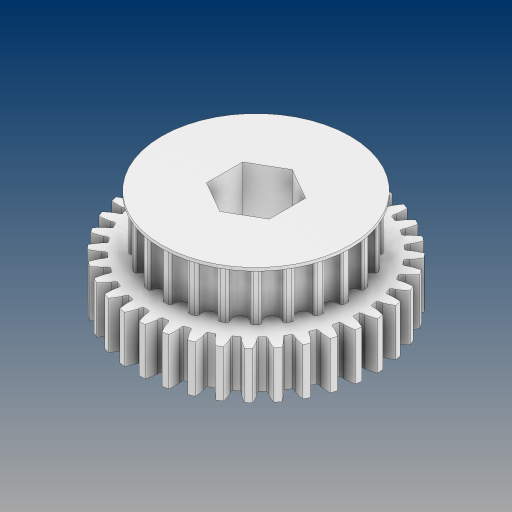
# Autodesk Inventor part: SHOT_005_36TGear-24TPulley
Saved by Autodesk Inventor 2024.3 (Build 283343000, 343)
## iProperties
Created: 2024-08-09
Part Number: SHOT_005_36TGear-24TPulley
Material: ABS Plastic
Document SubType Name: Modeling
Designer: Kenji
Density: 1.06 g/cm^3
Appearance: Smooth - White
Author: Kenji
Autodesk Inventor part; units mm, degrees
(part 1 of 2)
ref_plane "YZ Plane" through (0, 0, 0) normal (1, 0, 0) x (0, 1, 0)
ref_plane "XZ Plane" through (0, 0, 0) normal (0, 1, 0) x (-1, 0, 0)
ref_plane "XY Plane" through (0, 0, 0) normal (0, 0, 1) x (1, 0, 0)
sketch "Sketch1" plane through (0, 0, 0) normal (0, 1, 0) x (-1, 0, 0)
  circle A0 centre (0, 0) radius 22.86 construction
  circle A1 centre (0, 0) radius 24.13 construction
  line L0 (0, 0) -> (22.86, 0) construction
  line L1 (0, 0) -> (21.4269, 5.5414) construction
  line L2 (21.4269, 5.5414) -> (22.86, 0) construction
  arc A2 (21.4269, 5.5414) -> (20.1275, 9.2034) centre (0, 0) ccw construction
  arc A3 (22.1315, -0.1227) -> (21.4269, 5.5414) centre (0, 0) ccw construction
  line L3 (22.86, 0) -> (22.1315, -0.1227) construction
  line L4 (20.1275, 9.2034) -> (24.1256, 0.4597) construction
  line L5 (21.2725, 11.3902) -> (21.2725, -11.3902) construction
  line L6 (22.1315, -0.1227) -> (21.2725, -0.3449) construction
  line L7 (23.1177, 6.9159) -> (18.5715, -15.4064) construction
  line L8 (22.1315, -0.1227) -> (21.6794, -0.1463) construction
  line L9 (21.6794, -0.1463) -> (21.2725, -0.3449) construction
  line L10 (23.4095, 5.8526) -> (17.8483, -16.2387) construction
  line L11 (22.1315, -0.1227) -> (21.9049, -0.1242) construction
  line L12 (21.9049, -0.1242) -> (21.6794, -0.1463) construction
  line L13 (22.6036, 8.4459) -> (19.5599, -14.1303) construction
  line L14 (21.6794, -0.1463) -> (21.4414, -0.1748) construction
  line L15 (21.4414, -0.1748) -> (21.2725, -0.3449) construction
  line L16 (0, 0) -> (21.255, -0.928) construction
  arc A4 (21.255, -0.928) -> (21.2725, -0.3449) centre (0, 0) ccw
  arc A5 (21.2216, -1.5105) -> (21.255, -0.928) centre (0, 0) ccw
  line L17 (24.1256, 0.4597) -> (22.86, 0) construction
  line L18 (22.86, 0) -> (22.1315, -0.1227) construction
  spline S0 degree 2 poles (24.1256, 0.4597) (22.86, 0) (22.1315, -0.1227) knots 1 1 1 2 2 2
  line L19 (22.1315, -0.1227) -> (21.9049, -0.1242) construction
  line L20 (21.9049, -0.1242) -> (21.6794, -0.1463) construction
  line L21 (21.6794, -0.1463) -> (21.4414, -0.1748) construction
  line L22 (21.4414, -0.1748) -> (21.2725, -0.3449) construction
  spline S1 degree 4 poles (22.1315, -0.1227) (21.9049, -0.1242) (21.6794, -0.1463) (21.4414, -0.1748) (21.2725, -0.3449) knots 1 1 1 1 1 2 2 2 2 2
  arc A6 (21.2216, -1.5105) -> (21.255, -0.928) centre (0, 0) ccw
  line L23 (23.9937, -2.5606) -> (22.773, -1.9924) construction
  line L24 (22.773, -1.9924) -> (22.058, -1.8066) construction
  spline S2 degree 2 poles (23.9937, -2.5606) (22.773, -1.9924) (22.058, -1.8066) knots 1 1 1 2 2 2
  line L25 (22.058, -1.8066) -> (21.8324, -1.7854) construction
  line L26 (21.8324, -1.7854) -> (21.6096, -1.7437) construction
  line L27 (21.6096, -1.7437) -> (21.375, -1.6946) construction
  line L28 (21.375, -1.6946) -> (21.2216, -1.5105) construction
  spline S3 degree 4 poles (22.058, -1.8066) (21.8324, -1.7854) (21.6096, -1.7437) (21.375, -1.6946) (21.2216, -1.5105) knots 1 1 1 1 1 2 2 2 2 2
  line L29 (23.6793, 4.6421) -> (22.5127, 3.9696) construction
  spline S4 degree 2 poles (23.6793, 4.6421) (22.5127, 3.9696) (21.8166, 3.7222) knots 1 1 1 2 2 2
  line L30 (22.5127, 3.9696) -> (21.8166, 3.7222) construction
  spline S5 degree 2 poles (24.0739, 1.6447) (22.773, 1.9924) (22.0366, 2.0511) knots 1 1 1 2 2 2
  line L31 (24.0739, 1.6447) -> (22.773, 1.9924) construction
  line L32 (22.773, 1.9924) -> (22.0366, 2.0511) construction
  line L33 (22.0366, 2.0511) -> (21.8107, 2.0328) construction
  spline S6 degree 4 poles (22.0366, 2.0511) (21.8107, 2.0328) (21.5841, 2.0352) (21.3446, 2.0429) (21.1615, 2.1976) knots 1 1 1 1 1 2 2 2 2 2
  line L34 (21.8107, 2.0328) -> (21.5841, 2.0352) construction
  line L35 (21.5841, 2.0352) -> (21.3446, 2.0429) construction
  line L36 (21.3446, 2.0429) -> (21.1615, 2.1976) construction
  arc A7 (21.1615, 2.1976) -> (21.0933, 2.777) centre (0, 0) ccw
  arc A8 (21.0933, 2.777) -> (21.0092, 3.3543) centre (0, 0) ccw
  spline S7 degree 4 poles (21.8166, 3.7222) (21.5937, 3.6815) (21.3754, 3.6205) (21.146, 3.5511) (21.0092, 3.3543) knots 1 1 1 1 1 2 2 2 2 2
  line L37 (21.8166, 3.7222) -> (21.5937, 3.6815) construction
  line L38 (21.5937, 3.6815) -> (21.3754, 3.6205) construction
  line L39 (21.3754, 3.6205) -> (21.146, 3.5511) construction
  line L40 (21.146, 3.5511) -> (21.0092, 3.3543) construction
  line L41 (22.5134, 8.6834) -> (21.4814, 7.8186) construction
  spline S8 degree 2 poles (22.5134, 8.6834) (21.4814, 7.8186) (20.8388, 7.4541) knots 1 1 1 2 2 2
  line L42 (21.4814, 7.8186) -> (20.8388, 7.4541) construction
  spline S9 degree 2 poles (23.4225, 5.8001) (22.0811, 5.9166) (21.3456, 5.8466) knots 1 1 1 2 2 2
  line L43 (23.4225, 5.8001) -> (22.0811, 5.9166) construction
  line L44 (22.0811, 5.9166) -> (21.3456, 5.8466) construction
  line L45 (21.3456, 5.8466) -> (21.1264, 5.7894) construction
  spline S10 degree 4 poles (21.3456, 5.8466) (21.1264, 5.7894) (20.9028, 5.7524) (20.6656, 5.7183) (20.4584, 5.8389) knots 1 1 1 1 1 2 2 2 2 2
  line L46 (21.1264, 5.7894) -> (20.9028, 5.7524) construction
  line L47 (20.9028, 5.7524) -> (20.6656, 5.7183) construction
  line L48 (20.6656, 5.7183) -> (20.4584, 5.8389) construction
  arc A9 (20.4584, 5.8389) -> (20.2906, 6.3976) centre (0, 0) ccw
  arc A10 (20.2906, 6.3976) -> (20.1076, 6.9515) centre (0, 0) ccw
  spline S11 degree 4 poles (20.8388, 7.4541) (20.6264, 7.3752) (20.422, 7.2773) (20.2081, 7.1691) (20.1076, 6.9515) knots 1 1 1 1 1 2 2 2 2 2
  line L49 (20.8388, 7.4541) -> (20.6264, 7.3752) construction
  line L50 (20.6264, 7.3752) -> (20.422, 7.2773) construction
  line L51 (20.422, 7.2773) -> (20.2081, 7.1691) construction
  line L52 (20.2081, 7.1691) -> (20.1076, 6.9515) construction
  line L53 (20.6635, 12.4609) -> (19.7973, 11.43) construction
  spline S12 degree 2 poles (20.6635, 12.4609) (19.7973, 11.43) (19.2278, 10.9595) knots 1 1 1 2 2 2
  line L54 (19.7973, 11.43) -> (19.2278, 10.9595) construction
  spline S13 degree 2 poles (22.0595, 9.7793) (20.7182, 9.6611) (20.0061, 9.4644) knots 1 1 1 2 2 2
  line L55 (22.0595, 9.7793) -> (20.7182, 9.6611) construction
  line L56 (20.7182, 9.6611) -> (20.0061, 9.4644) construction
  line L57 (20.0061, 9.4644) -> (19.8001, 9.37) construction
  spline S14 degree 4 poles (20.0061, 9.4644) (19.8001, 9.37) (19.5864, 9.2947) (19.3586, 9.2199) (19.1337, 9.3027) knots 1 1 1 1 1 2 2 2 2 2
  line L58 (19.8001, 9.37) -> (19.5864, 9.2947) construction
  line L59 (19.5864, 9.2947) -> (19.3586, 9.2199) construction
  line L60 (19.3586, 9.2199) -> (19.1337, 9.3027) construction
  arc A11 (19.1337, 9.3027) -> (18.8714, 9.8238) centre (0, 0) ccw
  arc A12 (18.8714, 9.8238) -> (18.595, 10.3376) centre (0, 0) ccw
  spline S15 degree 4 poles (19.2278, 10.9595) (19.0323, 10.8449) (18.8481, 10.713) (18.6562, 10.5693) (18.595, 10.3376) knots 1 1 1 1 1 2 2 2 2 2
  line L61 (19.2278, 10.9595) -> (19.0323, 10.8449) construction
  line L62 (19.0323, 10.8449) -> (18.8481, 10.713) construction
  line L63 (18.8481, 10.713) -> (18.6562, 10.5693) construction
  line L64 (18.6562, 10.5693) -> (18.595, 10.3376) construction
  line L65 (18.1858, 15.8598) -> (17.5118, 14.6941) construction
  spline S16 degree 2 poles (18.1858, 15.8598) (17.5118, 14.6941) (17.0326, 14.1319) knots 1 1 1 2 2 2
  line L66 (17.5118, 14.6941) -> (17.0326, 14.1319) construction
  spline S17 degree 2 poles (20.0262, 13.4613) (18.7258, 13.112) (18.0587, 12.7946) knots 1 1 1 2 2 2
  line L67 (20.0262, 13.4613) -> (18.7258, 13.112) construction
  line L68 (18.7258, 13.112) -> (18.0587, 12.7946) construction
  line L69 (18.0587, 12.7946) -> (17.8722, 12.6659) construction
  spline S18 degree 4 poles (18.0587, 12.7946) (17.8722, 12.6659) (17.6748, 12.5546) (17.4635, 12.4415) (17.2276, 12.4839) knots 1 1 1 1 1 2 2 2 2 2
  line L70 (17.8722, 12.6659) -> (17.6748, 12.5546) construction
  line L71 (17.6748, 12.5546) -> (17.4635, 12.4415) construction
  line L72 (17.4635, 12.4415) -> (17.2276, 12.4839) construction
  arc A13 (17.2276, 12.4839) -> (16.8788, 12.9516) centre (0, 0) ccw
  arc A14 (16.8788, 12.9516) -> (16.5174, 13.4095) centre (0, 0) ccw
  spline S19 degree 4 poles (17.0326, 14.1319) (16.86, 13.9851) (16.7014, 13.8232) (16.5374, 13.6484) (16.5174, 13.4095) knots 1 1 1 1 1 2 2 2 2 2
  line L73 (17.0326, 14.1319) -> (16.86, 13.9851) construction
  line L74 (16.86, 13.9851) -> (16.7014, 13.8232) construction
  line L75 (16.7014, 13.8232) -> (16.5374, 13.6484) construction
  line L76 (16.5374, 13.6484) -> (16.5174, 13.4095) construction
  line L77 (15.1555, 18.7768) -> (14.6941, 17.5118) construction
  spline S20 degree 2 poles (15.1555, 18.7768) (14.6941, 17.5118) (14.3199, 16.8748) knots 1 1 1 2 2 2
  line L78 (14.6941, 17.5118) -> (14.3199, 16.8748) construction
  spline S21 degree 2 poles (17.3845, 16.7343) (16.1645, 16.1645) (15.5626, 15.7361) knots 1 1 1 2 2 2
  line L79 (17.3845, 16.7343) -> (16.1645, 16.1645) construction
  line L80 (16.1645, 16.1645) -> (15.5626, 15.7361) construction
  line L81 (15.5626, 15.7361) -> (15.4013, 15.5769) construction
  spline S22 degree 4 poles (15.5626, 15.7361) (15.4013, 15.5769) (15.2262, 15.4331) (15.0378, 15.2849) (14.7981, 15.2858) knots 1 1 1 1 1 2 2 2 2 2
  line L82 (15.4013, 15.5769) -> (15.2262, 15.4331) construction
  line L83 (15.2262, 15.4331) -> (15.0378, 15.2849) construction
  line L84 (15.0378, 15.2849) -> (14.7981, 15.2858) construction
  arc A15 (14.7981, 15.2858) -> (14.3734, 15.6858) centre (0, 0) ccw
  arc A16 (14.3734, 15.6858) -> (13.9379, 16.074) centre (0, 0) ccw
  spline S23 degree 4 poles (14.3199, 16.8748) (14.1753, 16.7003) (14.0473, 16.5133) (13.9162, 16.3127) (13.9379, 16.074) knots 1 1 1 1 1 2 2 2 2 2
  line L85 (14.3199, 16.8748) -> (14.1753, 16.7003) construction
  line L86 (14.1753, 16.7003) -> (14.0473, 16.5133) construction
  line L87 (14.0473, 16.5133) -> (13.9162, 16.3127) construction
  line L88 (13.9162, 16.3127) -> (13.9379, 16.074) construction
  line L89 (11.6647, 21.1233) -> (11.43, 19.7973) construction
  spline S24 degree 2 poles (11.6647, 21.1233) (11.43, 19.7973) (11.172, 19.1051) knots 1 1 1 2 2 2
  line L90 (11.43, 19.7973) -> (11.172, 19.1051) construction
  spline S25 degree 2 poles (14.2145, 19.4989) (13.112, 18.7258) (12.5936, 18.1995) knots 1 1 1 2 2 2
  line L91 (14.2145, 19.4989) -> (13.112, 18.7258) construction
  line L92 (13.112, 18.7258) -> (12.5936, 18.1995) construction
  line L93 (12.5936, 18.1995) -> (12.4624, 18.0147) construction
  spline S26 degree 4 poles (12.5936, 18.1995) (12.4624, 18.0147) (12.3149, 17.8426) (12.1551, 17.664) (11.9189, 17.6232) knots 1 1 1 1 1 2 2 2 2 2
  line L94 (12.4624, 18.0147) -> (12.3149, 17.8426) construction
  line L95 (12.3149, 17.8426) -> (12.1551, 17.664) construction
  line L96 (12.1551, 17.664) -> (11.9189, 17.6232) construction
  arc A17 (11.9189, 17.6232) -> (11.4312, 17.9434) centre (0, 0) ccw
  arc A18 (11.4312, 17.9434) -> (10.9349, 18.2501) centre (0, 0) ccw
  spline S27 degree 4 poles (11.172, 19.1051) (11.06, 18.9081) (10.9664, 18.7017) (10.8721, 18.4814) (10.9349, 18.2501) knots 1 1 1 1 1 2 2 2 2 2
  line L97 (11.172, 19.1051) -> (11.06, 18.9081) construction
  line L98 (11.06, 18.9081) -> (10.9664, 18.7017) construction
  line L99 (10.9664, 18.7017) -> (10.8721, 18.4814) construction
  line L100 (10.8721, 18.4814) -> (10.9349, 18.2501) construction
  line L101 (7.8195, 22.8279) -> (7.8186, 21.4814) construction
  spline S28 degree 2 poles (7.8195, 22.8279) (7.8186, 21.4814) (7.6847, 20.7548) knots 1 1 1 2 2 2
  line L102 (7.8186, 21.4814) -> (7.6847, 20.7548) construction
  spline S29 degree 2 poles (10.6126, 21.671) (9.6611, 20.7182) (9.242, 20.1098) knots 1 1 1 2 2 2
  line L103 (10.6126, 21.671) -> (9.6611, 20.7182) construction
  line L104 (9.6611, 20.7182) -> (9.242, 20.1098) construction
  line L105 (9.242, 20.1098) -> (9.1449, 19.9051) construction
  spline S30 degree 4 poles (9.242, 20.1098) (9.1449, 19.9051) (9.0295, 19.71) (8.9031, 19.5064) (8.6776, 19.4252) knots 1 1 1 1 1 2 2 2 2 2
  line L106 (9.1449, 19.9051) -> (9.0295, 19.71) construction
  line L107 (9.0295, 19.71) -> (8.9031, 19.5064) construction
  line L108 (8.9031, 19.5064) -> (8.6776, 19.4252) construction
  arc A19 (8.6776, 19.4252) -> (8.1417, 19.6558) centre (0, 0) ccw
  arc A20 (8.1417, 19.6558) -> (7.5997, 19.8717) centre (0, 0) ccw
  spline S31 degree 4 poles (7.6847, 20.7548) (7.6086, 20.5414) (7.5523, 20.3219) (7.4976, 20.0885) (7.5997, 19.8717) knots 1 1 1 1 1 2 2 2 2 2
  line L109 (7.6847, 20.7548) -> (7.6086, 20.5414) construction
  line L110 (7.6086, 20.5414) -> (7.5523, 20.3219) construction
  line L111 (7.5523, 20.3219) -> (7.4976, 20.0885) construction
  line L112 (7.4976, 20.0885) -> (7.5997, 19.8717) construction
  line L113 (3.7366, 23.8389) -> (3.9696, 22.5127) construction
  spline S32 degree 2 poles (3.7366, 23.8389) (3.9696, 22.5127) (3.9639, 21.774) knots 1 1 1 2 2 2
  line L114 (3.9696, 22.5127) -> (3.9639, 21.774) construction
  spline S33 degree 2 poles (6.6882, 23.1846) (5.9166, 22.0811) (5.6095, 21.4092) knots 1 1 1 2 2 2
  line L115 (6.6882, 23.1846) -> (5.9166, 22.0811) construction
  line L116 (5.9166, 22.0811) -> (5.6095, 21.4092) construction
  line L117 (5.6095, 21.4092) -> (5.5495, 21.1907) construction
  spline S34 degree 4 poles (5.6095, 21.4092) (5.5495, 21.1907) (5.4697, 20.9785) (5.3806, 20.756) (5.1726, 20.6369) knots 1 1 1 1 1 2 2 2 2 2
  line L118 (5.5495, 21.1907) -> (5.4697, 20.9785) construction
  line L119 (5.4697, 20.9785) -> (5.3806, 20.756) construction
  line L120 (5.3806, 20.756) -> (5.1726, 20.6369) construction
  arc A21 (5.1726, 20.6369) -> (4.6048, 20.771) centre (0, 0) ccw
  arc A22 (4.6048, 20.771) -> (4.0336, 20.8894) centre (0, 0) ccw
  spline S35 degree 4 poles (3.9639, 21.774) (3.926, 21.5506) (3.9087, 21.3246) (3.8954, 21.0853) (4.0336, 20.8894) knots 1 1 1 1 1 2 2 2 2 2
  line L121 (3.9639, 21.774) -> (3.926, 21.5506) construction
  line L122 (3.926, 21.5506) -> (3.9087, 21.3246) construction
  line L123 (3.9087, 21.3246) -> (3.8954, 21.0853) construction
  line L124 (3.8954, 21.0853) -> (4.0336, 20.8894) construction
  line L125 (-0.4597, 24.1256) -> (0, 22.86) construction
  spline S36 degree 2 poles (-0.4597, 24.1256) (0, 22.86) (0.1227, 22.1315) knots 1 1 1 2 2 2
  line L126 (0, 22.86) -> (0.1227, 22.1315) construction
  spline S37 degree 2 poles (2.5606, 23.9937) (1.9924, 22.773) (1.8066, 22.058) knots 1 1 1 2 2 2
  line L127 (2.5606, 23.9937) -> (1.9924, 22.773) construction
  line L128 (1.9924, 22.773) -> (1.8066, 22.058) construction
  line L129 (1.8066, 22.058) -> (1.7854, 21.8324) construction
  spline S38 degree 4 poles (1.8066, 22.058) (1.7854, 21.8324) (1.7437, 21.6096) (1.6946, 21.375) (1.5105, 21.2216) knots 1 1 1 1 1 2 2 2 2 2
  line L130 (1.7854, 21.8324) -> (1.7437, 21.6096) construction
  line L131 (1.7437, 21.6096) -> (1.6946, 21.375) construction
  line L132 (1.6946, 21.375) -> (1.5105, 21.2216) construction
  arc A23 (1.5105, 21.2216) -> (0.928, 21.255) centre (0, 0) ccw
  arc A24 (0.928, 21.255) -> (0.3449, 21.2725) centre (0, 0) ccw
  spline S39 degree 4 poles (0.1227, 22.1315) (0.1242, 21.9049) (0.1463, 21.6794) (0.1748, 21.4414) (0.3449, 21.2725) knots 1 1 1 1 1 2 2 2 2 2
  line L133 (0.1227, 22.1315) -> (0.1242, 21.9049) construction
  line L134 (0.1242, 21.9049) -> (0.1463, 21.6794) construction
  line L135 (0.1463, 21.6794) -> (0.1748, 21.4414) construction
  line L136 (0.1748, 21.4414) -> (0.3449, 21.2725) construction
  line L137 (-4.6421, 23.6793) -> (-3.9696, 22.5127) construction
  spline S40 degree 2 poles (-4.6421, 23.6793) (-3.9696, 22.5127) (-3.7222, 21.8166) knots 1 1 1 2 2 2
  line L138 (-3.9696, 22.5127) -> (-3.7222, 21.8166) construction
  spline S41 degree 2 poles (-1.6447, 24.0739) (-1.9924, 22.773) (-2.0511, 22.0366) knots 1 1 1 2 2 2
  line L139 (-1.6447, 24.0739) -> (-1.9924, 22.773) construction
  line L140 (-1.9924, 22.773) -> (-2.0511, 22.0366) construction
  line L141 (-2.0511, 22.0366) -> (-2.0328, 21.8107) construction
  spline S42 degree 4 poles (-2.0511, 22.0366) (-2.0328, 21.8107) (-2.0352, 21.5841) (-2.0429, 21.3446) (-2.1976, 21.1615) knots 1 1 1 1 1 2 2 2 2 2
  line L142 (-2.0328, 21.8107) -> (-2.0352, 21.5841) construction
  line L143 (-2.0352, 21.5841) -> (-2.0429, 21.3446) construction
  line L144 (-2.0429, 21.3446) -> (-2.1976, 21.1615) construction
  arc A25 (-2.1976, 21.1615) -> (-2.777, 21.0933) centre (0, 0) ccw
  arc A26 (-2.777, 21.0933) -> (-3.3543, 21.0092) centre (0, 0) ccw
  spline S43 degree 4 poles (-3.7222, 21.8166) (-3.6815, 21.5937) (-3.6205, 21.3754) (-3.5511, 21.146) (-3.3543, 21.0092) knots 1 1 1 1 1 2 2 2 2 2
  line L145 (-3.7222, 21.8166) -> (-3.6815, 21.5937) construction
  line L146 (-3.6815, 21.5937) -> (-3.6205, 21.3754) construction
  line L147 (-3.6205, 21.3754) -> (-3.5511, 21.146) construction
  line L148 (-3.5511, 21.146) -> (-3.3543, 21.0092) construction
  line L149 (-8.6834, 22.5134) -> (-7.8186, 21.4814) construction
  spline S44 degree 2 poles (-8.6834, 22.5134) (-7.8186, 21.4814) (-7.4541, 20.8388) knots 1 1 1 2 2 2
  line L150 (-7.8186, 21.4814) -> (-7.4541, 20.8388) construction
  spline S45 degree 2 poles (-5.8001, 23.4225) (-5.9166, 22.0811) (-5.8466, 21.3456) knots 1 1 1 2 2 2
  line L151 (-5.8001, 23.4225) -> (-5.9166, 22.0811) construction
  line L152 (-5.9166, 22.0811) -> (-5.8466, 21.3456) construction
  line L153 (-5.8466, 21.3456) -> (-5.7894, 21.1264) construction
  spline S46 degree 4 poles (-5.8466, 21.3456) (-5.7894, 21.1264) (-5.7524, 20.9028) (-5.7183, 20.6656) (-5.8389, 20.4584) knots 1 1 1 1 1 2 2 2 2 2
  line L154 (-5.7894, 21.1264) -> (-5.7524, 20.9028) construction
  line L155 (-5.7524, 20.9028) -> (-5.7183, 20.6656) construction
  line L156 (-5.7183, 20.6656) -> (-5.8389, 20.4584) construction
  arc A27 (-5.8389, 20.4584) -> (-6.3976, 20.2906) centre (0, 0) ccw
  arc A28 (-6.3976, 20.2906) -> (-6.9515, 20.1076) centre (0, 0) ccw
  spline S47 degree 4 poles (-7.4541, 20.8388) (-7.3752, 20.6264) (-7.2773, 20.422) (-7.1691, 20.2081) (-6.9515, 20.1076) knots 1 1 1 1 1 2 2 2 2 2
  line L157 (-7.4541, 20.8388) -> (-7.3752, 20.6264) construction
  line L158 (-7.3752, 20.6264) -> (-7.2773, 20.422) construction
  line L159 (-7.2773, 20.422) -> (-7.1691, 20.2081) construction
  line L160 (-7.1691, 20.2081) -> (-6.9515, 20.1076) construction
  line L161 (-12.4609, 20.6635) -> (-11.43, 19.7973) construction
  spline S48 degree 2 poles (-12.4609, 20.6635) (-11.43, 19.7973) (-10.9595, 19.2278) knots 1 1 1 2 2 2
  line L162 (-11.43, 19.7973) -> (-10.9595, 19.2278) construction
  spline S49 degree 2 poles (-9.7793, 22.0595) (-9.6611, 20.7182) (-9.4644, 20.0061) knots 1 1 1 2 2 2
  line L163 (-9.7793, 22.0595) -> (-9.6611, 20.7182) construction
  line L164 (-9.6611, 20.7182) -> (-9.4644, 20.0061) construction
  line L165 (-9.4644, 20.0061) -> (-9.37, 19.8001) construction
  spline S50 degree 4 poles (-9.4644, 20.0061) (-9.37, 19.8001) (-9.2947, 19.5864) (-9.2199, 19.3586) (-9.3027, 19.1337) knots 1 1 1 1 1 2 2 2 2 2
  line L166 (-9.37, 19.8001) -> (-9.2947, 19.5864) construction
  line L167 (-9.2947, 19.5864) -> (-9.2199, 19.3586) construction
  line L168 (-9.2199, 19.3586) -> (-9.3027, 19.1337) construction
  arc A29 (-9.3027, 19.1337) -> (-9.8238, 18.8714) centre (0, 0) ccw
  arc A30 (-9.8238, 18.8714) -> (-10.3376, 18.595) centre (0, 0) ccw
  spline S51 degree 4 poles (-10.9595, 19.2278) (-10.8449, 19.0323) (-10.713, 18.8481) (-10.5693, 18.6562) (-10.3376, 18.595) knots 1 1 1 1 1 2 2 2 2 2
  line L169 (-10.9595, 19.2278) -> (-10.8449, 19.0323) construction
  line L170 (-10.8449, 19.0323) -> (-10.713, 18.8481) construction
  line L171 (-10.713, 18.8481) -> (-10.5693, 18.6562) construction
  line L172 (-10.5693, 18.6562) -> (-10.3376, 18.595) construction
  line L173 (-15.8598, 18.1858) -> (-14.6941, 17.5118) construction
  spline S52 degree 2 poles (-15.8598, 18.1858) (-14.6941, 17.5118) (-14.1319, 17.0326) knots 1 1 1 2 2 2
  line L174 (-14.6941, 17.5118) -> (-14.1319, 17.0326) construction
  spline S53 degree 2 poles (-13.4613, 20.0262) (-13.112, 18.7258) (-12.7946, 18.0587) knots 1 1 1 2 2 2
  line L175 (-13.4613, 20.0262) -> (-13.112, 18.7258) construction
  line L176 (-13.112, 18.7258) -> (-12.7946, 18.0587) construction
  line L177 (-12.7946, 18.0587) -> (-12.6659, 17.8722) construction
  spline S54 degree 4 poles (-12.7946, 18.0587) (-12.6659, 17.8722) (-12.5546, 17.6748) (-12.4415, 17.4635) (-12.4839, 17.2276) knots 1 1 1 1 1 2 2 2 2 2
  line L178 (-12.6659, 17.8722) -> (-12.5546, 17.6748) construction
  line L179 (-12.5546, 17.6748) -> (-12.4415, 17.4635) construction
  line L180 (-12.4415, 17.4635) -> (-12.4839, 17.2276) construction
  arc A31 (-12.4839, 17.2276) -> (-12.9516, 16.8788) centre (0, 0) ccw
  arc A32 (-12.9516, 16.8788) -> (-13.4095, 16.5174) centre (0, 0) ccw
  spline S55 degree 4 poles (-14.1319, 17.0326) (-13.9851, 16.86) (-13.8232, 16.7014) (-13.6484, 16.5374) (-13.4095, 16.5174) knots 1 1 1 1 1 2 2 2 2 2
  line L181 (-14.1319, 17.0326) -> (-13.9851, 16.86) construction
  line L182 (-13.9851, 16.86) -> (-13.8232, 16.7014) construction
  line L183 (-13.8232, 16.7014) -> (-13.6484, 16.5374) construction
  line L184 (-13.6484, 16.5374) -> (-13.4095, 16.5174) construction
  line L185 (-18.7768, 15.1555) -> (-17.5118, 14.6941) construction
  spline S56 degree 2 poles (-18.7768, 15.1555) (-17.5118, 14.6941) (-16.8748, 14.3199) knots 1 1 1 2 2 2
  line L186 (-17.5118, 14.6941) -> (-16.8748, 14.3199) construction
  spline S57 degree 2 poles (-16.7343, 17.3845) (-16.1645, 16.1645) (-15.7361, 15.5626) knots 1 1 1 2 2 2
  line L187 (-16.7343, 17.3845) -> (-16.1645, 16.1645) construction
  line L188 (-16.1645, 16.1645) -> (-15.7361, 15.5626) construction
  line L189 (-15.7361, 15.5626) -> (-15.5769, 15.4013) construction
  spline S58 degree 4 poles (-15.7361, 15.5626) (-15.5769, 15.4013) (-15.4331, 15.2262) (-15.2849, 15.0378) (-15.2858, 14.7981) knots 1 1 1 1 1 2 2 2 2 2
  line L190 (-15.5769, 15.4013) -> (-15.4331, 15.2262) construction
  line L191 (-15.4331, 15.2262) -> (-15.2849, 15.0378) construction
  line L192 (-15.2849, 15.0378) -> (-15.2858, 14.7981) construction
  arc A33 (-15.2858, 14.7981) -> (-15.6858, 14.3734) centre (0, 0) ccw
  arc A34 (-15.6858, 14.3734) -> (-16.074, 13.9379) centre (0, 0) ccw
  spline S59 degree 4 poles (-16.8748, 14.3199) (-16.7003, 14.1753) (-16.5133, 14.0473) (-16.3127, 13.9162) (-16.074, 13.9379) knots 1 1 1 1 1 2 2 2 2 2
  line L193 (-16.8748, 14.3199) -> (-16.7003, 14.1753) construction
  line L194 (-16.7003, 14.1753) -> (-16.5133, 14.0473) construction
  line L195 (-16.5133, 14.0473) -> (-16.3127, 13.9162) construction
  line L196 (-16.3127, 13.9162) -> (-16.074, 13.9379) construction
  line L197 (-21.1233, 11.6647) -> (-19.7973, 11.43) construction
  spline S60 degree 2 poles (-21.1233, 11.6647) (-19.7973, 11.43) (-19.1051, 11.172) knots 1 1 1 2 2 2
  line L198 (-19.7973, 11.43) -> (-19.1051, 11.172) construction
  spline S61 degree 2 poles (-19.4989, 14.2145) (-18.7258, 13.112) (-18.1995, 12.5936) knots 1 1 1 2 2 2
  line L199 (-19.4989, 14.2145) -> (-18.7258, 13.112) construction
  line L200 (-18.7258, 13.112) -> (-18.1995, 12.5936) construction
  line L201 (-18.1995, 12.5936) -> (-18.0147, 12.4624) construction
  spline S62 degree 4 poles (-18.1995, 12.5936) (-18.0147, 12.4624) (-17.8426, 12.3149) (-17.664, 12.1551) (-17.6232, 11.9189) knots 1 1 1 1 1 2 2 2 2 2
  line L202 (-18.0147, 12.4624) -> (-17.8426, 12.3149) construction
  line L203 (-17.8426, 12.3149) -> (-17.664, 12.1551) construction
  line L204 (-17.664, 12.1551) -> (-17.6232, 11.9189) construction
  arc A35 (-17.6232, 11.9189) -> (-17.9434, 11.4312) centre (0, 0) ccw
  arc A36 (-17.9434, 11.4312) -> (-18.2501, 10.9349) centre (0, 0) ccw
  spline S63 degree 4 poles (-19.1051, 11.172) (-18.9081, 11.06) (-18.7017, 10.9664) (-18.4814, 10.8721) (-18.2501, 10.9349) knots 1 1 1 1 1 2 2 2 2 2
  line L205 (-19.1051, 11.172) -> (-18.9081, 11.06) construction
  line L206 (-18.9081, 11.06) -> (-18.7017, 10.9664) construction
  line L207 (-18.7017, 10.9664) -> (-18.4814, 10.8721) construction
  line L208 (-18.4814, 10.8721) -> (-18.2501, 10.9349) construction
  line L209 (-22.8279, 7.8195) -> (-21.4814, 7.8186) construction
  spline S64 degree 2 poles (-22.8279, 7.8195) (-21.4814, 7.8186) (-20.7548, 7.6847) knots 1 1 1 2 2 2
  line L210 (-21.4814, 7.8186) -> (-20.7548, 7.6847) construction
  spline S65 degree 2 poles (-21.671, 10.6126) (-20.7182, 9.6611) (-20.1098, 9.242) knots 1 1 1 2 2 2
  line L211 (-21.671, 10.6126) -> (-20.7182, 9.6611) construction
  line L212 (-20.7182, 9.6611) -> (-20.1098, 9.242) construction
  line L213 (-20.1098, 9.242) -> (-19.9051, 9.1449) construction
  spline S66 degree 4 poles (-20.1098, 9.242) (-19.9051, 9.1449) (-19.71, 9.0295) (-19.5064, 8.9031) (-19.4252, 8.6776) knots 1 1 1 1 1 2 2 2 2 2
  line L214 (-19.9051, 9.1449) -> (-19.71, 9.0295) construction
  line L215 (-19.71, 9.0295) -> (-19.5064, 8.9031) construction
  line L216 (-19.5064, 8.9031) -> (-19.4252, 8.6776) construction
  arc A37 (-19.4252, 8.6776) -> (-19.6558, 8.1417) centre (0, 0) ccw
  arc A38 (-19.6558, 8.1417) -> (-19.8717, 7.5997) centre (0, 0) ccw
  spline S67 degree 4 poles (-20.7548, 7.6847) (-20.5414, 7.6086) (-20.3219, 7.5523) (-20.0885, 7.4976) (-19.8717, 7.5997) knots 1 1 1 1 1 2 2 2 2 2
  line L217 (-20.7548, 7.6847) -> (-20.5414, 7.6086) construction
  line L218 (-20.5414, 7.6086) -> (-20.3219, 7.5523) construction
  line L219 (-20.3219, 7.5523) -> (-20.0885, 7.4976) construction
  line L220 (-20.0885, 7.4976) -> (-19.8717, 7.5997) construction
  line L221 (-23.8389, 3.7366) -> (-22.5127, 3.9696) construction
  spline S68 degree 2 poles (-23.8389, 3.7366) (-22.5127, 3.9696) (-21.774, 3.9639) knots 1 1 1 2 2 2
  line L222 (-22.5127, 3.9696) -> (-21.774, 3.9639) construction
  spline S69 degree 2 poles (-23.1846, 6.6882) (-22.0811, 5.9166) (-21.4092, 5.6095) knots 1 1 1 2 2 2
  line L223 (-23.1846, 6.6882) -> (-22.0811, 5.9166) construction
  line L224 (-22.0811, 5.9166) -> (-21.4092, 5.6095) construction
  line L225 (-21.4092, 5.6095) -> (-21.1907, 5.5495) construction
  spline S70 degree 4 poles (-21.4092, 5.6095) (-21.1907, 5.5495) (-20.9785, 5.4697) (-20.756, 5.3806) (-20.6369, 5.1726) knots 1 1 1 1 1 2 2 2 2 2
  line L226 (-21.1907, 5.5495) -> (-20.9785, 5.4697) construction
  line L227 (-20.9785, 5.4697) -> (-20.756, 5.3806) construction
  line L228 (-20.756, 5.3806) -> (-20.6369, 5.1726) construction
  arc A39 (-20.6369, 5.1726) -> (-20.771, 4.6048) centre (0, 0) ccw
  arc A40 (-20.771, 4.6048) -> (-20.8894, 4.0336) centre (0, 0) ccw
  spline S71 degree 4 poles (-21.774, 3.9639) (-21.5506, 3.926) (-21.3246, 3.9087) (-21.0853, 3.8954) (-20.8894, 4.0336) knots 1 1 1 1 1 2 2 2 2 2
  line L229 (-21.774, 3.9639) -> (-21.5506, 3.926) construction
  line L230 (-21.5506, 3.926) -> (-21.3246, 3.9087) construction
  line L231 (-21.3246, 3.9087) -> (-21.0853, 3.8954) construction
  line L232 (-21.0853, 3.8954) -> (-20.8894, 4.0336) construction
  line L233 (-24.1256, -0.4597) -> (-22.86, 0) construction
  spline S72 degree 2 poles (-24.1256, -0.4597) (-22.86, 0) (-22.1315, 0.1227) knots 1 1 1 2 2 2
  line L234 (-22.86, 0) -> (-22.1315, 0.1227) construction
  spline S73 degree 2 poles (-23.9937, 2.5606) (-22.773, 1.9924) (-22.058, 1.8066) knots 1 1 1 2 2 2
  line L235 (-23.9937, 2.5606) -> (-22.773, 1.9924) construction
  line L236 (-22.773, 1.9924) -> (-22.058, 1.8066) construction
  line L237 (-22.058, 1.8066) -> (-21.8324, 1.7854) construction
  spline S74 degree 4 poles (-22.058, 1.8066) (-21.8324, 1.7854) (-21.6096, 1.7437) (-21.375, 1.6946) (-21.2216, 1.5105) knots 1 1 1 1 1 2 2 2 2 2
  line L238 (-21.8324, 1.7854) -> (-21.6096, 1.7437) construction
  line L239 (-21.6096, 1.7437) -> (-21.375, 1.6946) construction
  line L240 (-21.375, 1.6946) -> (-21.2216, 1.5105) construction
  arc A41 (-21.2216, 1.5105) -> (-21.255, 0.928) centre (0, 0) ccw
  arc A42 (-21.255, 0.928) -> (-21.2725, 0.3449) centre (0, 0) ccw
  spline S75 degree 4 poles (-22.1315, 0.1227) (-21.9049, 0.1242) (-21.6794, 0.1463) (-21.4414, 0.1748) (-21.2725, 0.3449) knots 1 1 1 1 1 2 2 2 2 2
  line L241 (-22.1315, 0.1227) -> (-21.9049, 0.1242) construction
  line L242 (-21.9049, 0.1242) -> (-21.6794, 0.1463) construction
  line L243 (-21.6794, 0.1463) -> (-21.4414, 0.1748) construction
  line L244 (-21.4414, 0.1748) -> (-21.2725, 0.3449) construction
  line L245 (-23.6793, -4.6421) -> (-22.5127, -3.9696) construction
  spline S76 degree 2 poles (-23.6793, -4.6421) (-22.5127, -3.9696) (-21.8166, -3.7222) knots 1 1 1 2 2 2
  line L246 (-22.5127, -3.9696) -> (-21.8166, -3.7222) construction
  spline S77 degree 2 poles (-24.0739, -1.6447) (-22.773, -1.9924) (-22.0366, -2.0511) knots 1 1 1 2 2 2
  line L247 (-24.0739, -1.6447) -> (-22.773, -1.9924) construction
  line L248 (-22.773, -1.9924) -> (-22.0366, -2.0511) construction
  line L249 (-22.0366, -2.0511) -> (-21.8107, -2.0328) construction
  spline S78 degree 4 poles (-22.0366, -2.0511) (-21.8107, -2.0328) (-21.5841, -2.0352) (-21.3446, -2.0429) (-21.1615, -2.1976) knots 1 1 1 1 1 2 2 2 2 2
  line L250 (-21.8107, -2.0328) -> (-21.5841, -2.0352) construction
  line L251 (-21.5841, -2.0352) -> (-21.3446, -2.0429) construction
  line L252 (-21.3446, -2.0429) -> (-21.1615, -2.1976) construction
  arc A43 (-21.1615, -2.1976) -> (-21.0933, -2.777) centre (0, 0) ccw
  arc A44 (-21.0933, -2.777) -> (-21.0092, -3.3543) centre (0, 0) ccw
  spline S79 degree 4 poles (-21.8166, -3.7222) (-21.5937, -3.6815) (-21.3754, -3.6205) (-21.146, -3.5511) (-21.0092, -3.3543) knots 1 1 1 1 1 2 2 2 2 2
  line L253 (-21.8166, -3.7222) -> (-21.5937, -3.6815) construction
  line L254 (-21.5937, -3.6815) -> (-21.3754, -3.6205) construction
  line L255 (-21.3754, -3.6205) -> (-21.146, -3.5511) construction
  line L256 (-21.146, -3.5511) -> (-21.0092, -3.3543) construction
  line L257 (-22.5134, -8.6834) -> (-21.4814, -7.8186) construction
  spline S80 degree 2 poles (-22.5134, -8.6834) (-21.4814, -7.8186) (-20.8388, -7.4541) knots 1 1 1 2 2 2
  line L258 (-21.4814, -7.8186) -> (-20.8388, -7.4541) construction
  spline S81 degree 2 poles (-23.4225, -5.8001) (-22.0811, -5.9166) (-21.3456, -5.8466) knots 1 1 1 2 2 2
  line L259 (-23.4225, -5.8001) -> (-22.0811, -5.9166) construction
  line L260 (-22.0811, -5.9166) -> (-21.3456, -5.8466) construction
  line L261 (-21.3456, -5.8466) -> (-21.1264, -5.7894) construction
  spline S82 degree 4 poles (-21.3456, -5.8466) (-21.1264, -5.7894) (-20.9028, -5.7524) (-20.6656, -5.7183) (-20.4584, -5.8389) knots 1 1 1 1 1 2 2 2 2 2
  line L262 (-21.1264, -5.7894) -> (-20.9028, -5.7524) construction
  line L263 (-20.9028, -5.7524) -> (-20.6656, -5.7183) construction
  line L264 (-20.6656, -5.7183) -> (-20.4584, -5.8389) construction
  arc A45 (-20.4584, -5.8389) -> (-20.2906, -6.3976) centre (0, 0) ccw
  arc A46 (-20.2906, -6.3976) -> (-20.1076, -6.9515) centre (0, 0) ccw
  spline S83 degree 4 poles (-20.8388, -7.4541) (-20.6264, -7.3752) (-20.422, -7.2773) (-20.2081, -7.1691) (-20.1076, -6.9515) knots 1 1 1 1 1 2 2 2 2 2
  line L265 (-20.8388, -7.4541) -> (-20.6264, -7.3752) construction
  line L266 (-20.6264, -7.3752) -> (-20.422, -7.2773) construction
  line L267 (-20.422, -7.2773) -> (-20.2081, -7.1691) construction
  line L268 (-20.2081, -7.1691) -> (-20.1076, -6.9515) construction
  line L269 (-20.6635, -12.4609) -> (-19.7973, -11.43) construction
  spline S84 degree 2 poles (-20.6635, -12.4609) (-19.7973, -11.43) (-19.2278, -10.9595) knots 1 1 1 2 2 2
  line L270 (-19.7973, -11.43) -> (-19.2278, -10.9595) construction
  spline S85 degree 2 poles (-22.0595, -9.7793) (-20.7182, -9.6611) (-20.0061, -9.4644) knots 1 1 1 2 2 2
  line L271 (-22.0595, -9.7793) -> (-20.7182, -9.6611) construction
  line L272 (-20.7182, -9.6611) -> (-20.0061, -9.4644) construction
  line L273 (-20.0061, -9.4644) -> (-19.8001, -9.37) construction
  spline S86 degree 4 poles (-20.0061, -9.4644) (-19.8001, -9.37) (-19.5864, -9.2947) (-19.3586, -9.2199) (-19.1337, -9.3027) knots 1 1 1 1 1 2 2 2 2 2
  line L274 (-19.8001, -9.37) -> (-19.5864, -9.2947) construction
  line L275 (-19.5864, -9.2947) -> (-19.3586, -9.2199) construction
  line L276 (-19.3586, -9.2199) -> (-19.1337, -9.3027) construction
  arc A47 (-19.1337, -9.3027) -> (-18.8714, -9.8238) centre (0, 0) ccw
  arc A48 (-18.8714, -9.8238) -> (-18.595, -10.3376) centre (0, 0) ccw
  spline S87 degree 4 poles (-19.2278, -10.9595) (-19.0323, -10.8449) (-18.8481, -10.713) (-18.6562, -10.5693) (-18.595, -10.3376) knots 1 1 1 1 1 2 2 2 2 2
  line L277 (-19.2278, -10.9595) -> (-19.0323, -10.8449) construction
  line L278 (-19.0323, -10.8449) -> (-18.8481, -10.713) construction
  line L279 (-18.8481, -10.713) -> (-18.6562, -10.5693) construction
  line L280 (-18.6562, -10.5693) -> (-18.595, -10.3376) construction
  line L281 (-18.1858, -15.8598) -> (-17.5118, -14.6941) construction
  spline S88 degree 2 poles (-18.1858, -15.8598) (-17.5118, -14.6941) (-17.0326, -14.1319) knots 1 1 1 2 2 2
  line L282 (-17.5118, -14.6941) -> (-17.0326, -14.1319) construction
  spline S89 degree 2 poles (-20.0262, -13.4613) (-18.7258, -13.112) (-18.0587, -12.7946) knots 1 1 1 2 2 2
  line L283 (-20.0262, -13.4613) -> (-18.7258, -13.112) construction
  line L284 (-18.7258, -13.112) -> (-18.0587, -12.7946) construction
  line L285 (-18.0587, -12.7946) -> (-17.8722, -12.6659) construction
  spline S90 degree 4 poles (-18.0587, -12.7946) (-17.8722, -12.6659) (-17.6748, -12.5546) (-17.4635, -12.4415) (-17.2276, -12.4839) knots 1 1 1 1 1 2 2 2 2 2
  line L286 (-17.8722, -12.6659) -> (-17.6748, -12.5546) construction
  line L287 (-17.6748, -12.5546) -> (-17.4635, -12.4415) construction
  line L288 (-17.4635, -12.4415) -> (-17.2276, -12.4839) construction
  arc A49 (-17.2276, -12.4839) -> (-16.8788, -12.9516) centre (0, 0) ccw
  arc A50 (-16.8788, -12.9516) -> (-16.5174, -13.4095) centre (0, 0) ccw
  spline S91 degree 4 poles (-17.0326, -14.1319) (-16.86, -13.9851) (-16.7014, -13.8232) (-16.5374, -13.6484) (-16.5174, -13.4095) knots 1 1 1 1 1 2 2 2 2 2
  line L289 (-17.0326, -14.1319) -> (-16.86, -13.9851) construction
  line L290 (-16.86, -13.9851) -> (-16.7014, -13.8232) construction
  line L291 (-16.7014, -13.8232) -> (-16.5374, -13.6484) construction
  line L292 (-16.5374, -13.6484) -> (-16.5174, -13.4095) construction
  line L293 (-15.1555, -18.7768) -> (-14.6941, -17.5118) construction
  spline S92 degree 2 poles (-15.1555, -18.7768) (-14.6941, -17.5118) (-14.3199, -16.8748) knots 1 1 1 2 2 2
  line L294 (-14.6941, -17.5118) -> (-14.3199, -16.8748) construction
  spline S93 degree 2 poles (-17.3845, -16.7343) (-16.1645, -16.1645) (-15.5626, -15.7361) knots 1 1 1 2 2 2
  line L295 (-17.3845, -16.7343) -> (-16.1645, -16.1645) construction
  line L296 (-16.1645, -16.1645) -> (-15.5626, -15.7361) construction
  line L297 (-15.5626, -15.7361) -> (-15.4013, -15.5769) construction
  spline S94 degree 4 poles (-15.5626, -15.7361) (-15.4013, -15.5769) (-15.2262, -15.4331) (-15.0378, -15.2849) (-14.7981, -15.2858) knots 1 1 1 1 1 2 2 2 2 2
  line L298 (-15.4013, -15.5769) -> (-15.2262, -15.4331) construction
  line L299 (-15.2262, -15.4331) -> (-15.0378, -15.2849) construction
  line L300 (-15.0378, -15.2849) -> (-14.7981, -15.2858) construction
  arc A51 (-14.7981, -15.2858) -> (-14.3734, -15.6858) centre (0, 0) ccw
  arc A52 (-14.3734, -15.6858) -> (-13.9379, -16.074) centre (0, 0) ccw
  spline S95 degree 4 poles (-14.3199, -16.8748) (-14.1753, -16.7003) (-14.0473, -16.5133) (-13.9162, -16.3127) (-13.9379, -16.074) knots 1 1 1 1 1 2 2 2 2 2
  line L301 (-14.3199, -16.8748) -> (-14.1753, -16.7003) construction
  line L302 (-14.1753, -16.7003) -> (-14.0473, -16.5133) construction
  line L303 (-14.0473, -16.5133) -> (-13.9162, -16.3127) construction
  line L304 (-13.9162, -16.3127) -> (-13.9379, -16.074) construction
  line L305 (-11.6647, -21.1233) -> (-11.43, -19.7973) construction
  spline S96 degree 2 poles (-11.6647, -21.1233) (-11.43, -19.7973) (-11.172, -19.1051) knots 1 1 1 2 2 2
  line L306 (-11.43, -19.7973) -> (-11.172, -19.1051) construction
  spline S97 degree 2 poles (-14.2145, -19.4989) (-13.112, -18.7258) (-12.5936, -18.1995) knots 1 1 1 2 2 2
  line L307 (-14.2145, -19.4989) -> (-13.112, -18.7258) construction
  line L308 (-13.112, -18.7258) -> (-12.5936, -18.1995) construction
  line L309 (-12.5936, -18.1995) -> (-12.4624, -18.0147) construction
  spline S98 degree 4 poles (-12.5936, -18.1995) (-12.4624, -18.0147) (-12.3149, -17.8426) (-12.1551, -17.664) (-11.9189, -17.6232) knots 1 1 1 1 1 2 2 2 2 2
  line L310 (-12.4624, -18.0147) -> (-12.3149, -17.8426) construction
  line L311 (-12.3149, -17.8426) -> (-12.1551, -17.664) construction
  line L312 (-12.1551, -17.664) -> (-11.9189, -17.6232) construction
  arc A53 (-11.9189, -17.6232) -> (-11.4312, -17.9434) centre (0, 0) ccw
  arc A54 (-11.4312, -17.9434) -> (-10.9349, -18.2501) centre (0, 0) ccw
  spline S99 degree 4 poles (-11.172, -19.1051) (-11.06, -18.9081) (-10.9664, -18.7017) (-10.8721, -18.4814) (-10.9349, -18.2501) knots 1 1 1 1 1 2 2 2 2 2
  line L313 (-11.172, -19.1051) -> (-11.06, -18.9081) construction
  line L314 (-11.06, -18.9081) -> (-10.9664, -18.7017) construction
  line L315 (-10.9664, -18.7017) -> (-10.8721, -18.4814) construction
  line L316 (-10.8721, -18.4814) -> (-10.9349, -18.2501) construction
  line L317 (-7.8195, -22.8279) -> (-7.8186, -21.4814) construction
  spline S100 degree 2 poles (-7.8195, -22.8279) (-7.8186, -21.4814) (-7.6847, -20.7548) knots 1 1 1 2 2 2
  line L318 (-7.8186, -21.4814) -> (-7.6847, -20.7548) construction
  spline S101 degree 2 poles (-10.6126, -21.671) (-9.6611, -20.7182) (-9.242, -20.1098) knots 1 1 1 2 2 2
  line L319 (-10.6126, -21.671) -> (-9.6611, -20.7182) construction
  line L320 (-9.6611, -20.7182) -> (-9.242, -20.1098) construction
  line L321 (-9.242, -20.1098) -> (-9.1449, -19.9051) construction
  spline S102 degree 4 poles (-9.242, -20.1098) (-9.1449, -19.9051) (-9.0295, -19.71) (-8.9031, -19.5064) (-8.6776, -19.4252) knots 1 1 1 1 1 2 2 2 2 2
  line L322 (-9.1449, -19.9051) -> (-9.0295, -19.71) construction
  line L323 (-9.0295, -19.71) -> (-8.9031, -19.5064) construction
  line L324 (-8.9031, -19.5064) -> (-8.6776, -19.4252) construction
  arc A55 (-8.6776, -19.4252) -> (-8.1417, -19.6558) centre (0, 0) ccw
  arc A56 (-8.1417, -19.6558) -> (-7.5997, -19.8717) centre (0, 0) ccw
  spline S103 degree 4 poles (-7.6847, -20.7548) (-7.6086, -20.5414) (-7.5523, -20.3219) (-7.4976, -20.0885) (-7.5997, -19.8717) knots 1 1 1 1 1 2 2 2 2 2
  line L325 (-7.6847, -20.7548) -> (-7.6086, -20.5414) construction
  line L326 (-7.6086, -20.5414) -> (-7.5523, -20.3219) construction
  line L327 (-7.5523, -20.3219) -> (-7.4976, -20.0885) construction
  line L328 (-7.4976, -20.0885) -> (-7.5997, -19.8717) construction
  line L329 (-3.7366, -23.8389) -> (-3.9696, -22.5127) construction
  spline S104 degree 2 poles (-3.7366, -23.8389) (-3.9696, -22.5127) (-3.9639, -21.774) knots 1 1 1 2 2 2
  line L330 (-3.9696, -22.5127) -> (-3.9639, -21.774) construction
  spline S105 degree 2 poles (-6.6882, -23.1846) (-5.9166, -22.0811) (-5.6095, -21.4092) knots 1 1 1 2 2 2
  line L331 (-6.6882, -23.1846) -> (-5.9166, -22.0811) construction
  line L332 (-5.9166, -22.0811) -> (-5.6095, -21.4092) construction
  line L333 (-5.6095, -21.4092) -> (-5.5495, -21.1907) construction
  spline S106 degree 4 poles (-5.6095, -21.4092) (-5.5495, -21.1907) (-5.4697, -20.9785) (-5.3806, -20.756) (-5.1726, -20.6369) knots 1 1 1 1 1 2 2 2 2 2
  line L334 (-5.5495, -21.1907) -> (-5.4697, -20.9785) construction
  line L335 (-5.4697, -20.9785) -> (-5.3806, -20.756) construction
  line L336 (-5.3806, -20.756) -> (-5.1726, -20.6369) construction
  arc A57 (-5.1726, -20.6369) -> (-4.6048, -20.771) centre (0, 0) ccw
  arc A58 (-4.6048, -20.771) -> (-4.0336, -20.8894) centre (0, 0) ccw
  spline S107 degree 4 poles (-3.9639, -21.774) (-3.926, -21.5506) (-3.9087, -21.3246) (-3.8954, -21.0853) (-4.0336, -20.8894) knots 1 1 1 1 1 2 2 2 2 2
  line L337 (-3.9639, -21.774) -> (-3.926, -21.5506) construction
  line L338 (-3.926, -21.5506) -> (-3.9087, -21.3246) construction
  line L339 (-3.9087, -21.3246) -> (-3.8954, -21.0853) construction
  line L340 (-3.8954, -21.0853) -> (-4.0336, -20.8894) construction
  line L341 (0.4597, -24.1256) -> (0, -22.86) construction
  spline S108 degree 2 poles (0.4597, -24.1256) (0, -22.86) (-0.1227, -22.1315) knots 1 1 1 2 2 2
  line L342 (0, -22.86) -> (-0.1227, -22.1315) construction
  spline S109 degree 2 poles (-2.5606, -23.9937) (-1.9924, -22.773) (-1.8066, -22.058) knots 1 1 1 2 2 2
  line L343 (-2.5606, -23.9937) -> (-1.9924, -22.773) construction
  line L344 (-1.9924, -22.773) -> (-1.8066, -22.058) construction
  line L345 (-1.8066, -22.058) -> (-1.7854, -21.8324) construction
  spline S110 degree 4 poles (-1.8066, -22.058) (-1.7854, -21.8324) (-1.7437, -21.6096) (-1.6946, -21.375) (-1.5105, -21.2216) knots 1 1 1 1 1 2 2 2 2 2
  line L346 (-1.7854, -21.8324) -> (-1.7437, -21.6096) construction
  line L347 (-1.7437, -21.6096) -> (-1.6946, -21.375) construction
  line L348 (-1.6946, -21.375) -> (-1.5105, -21.2216) construction
  arc A59 (-1.5105, -21.2216) -> (-0.928, -21.255) centre (0, 0) ccw
  arc A60 (-0.928, -21.255) -> (-0.3449, -21.2725) centre (0, 0) ccw
  spline S111 degree 4 poles (-0.1227, -22.1315) (-0.1242, -21.9049) (-0.1463, -21.6794) (-0.1748, -21.4414) (-0.3449, -21.2725) knots 1 1 1 1 1 2 2 2 2 2
  line L349 (-0.1227, -22.1315) -> (-0.1242, -21.9049) construction
  line L350 (-0.1242, -21.9049) -> (-0.1463, -21.6794) construction
  line L351 (-0.1463, -21.6794) -> (-0.1748, -21.4414) construction
  line L352 (-0.1748, -21.4414) -> (-0.3449, -21.2725) construction
  line L353 (4.6421, -23.6793) -> (3.9696, -22.5127) construction
  spline S112 degree 2 poles (4.6421, -23.6793) (3.9696, -22.5127) (3.7222, -21.8166) knots 1 1 1 2 2 2
  line L354 (3.9696, -22.5127) -> (3.7222, -21.8166) construction
  spline S113 degree 2 poles (1.6447, -24.0739) (1.9924, -22.773) (2.0511, -22.0366) knots 1 1 1 2 2 2
  line L355 (1.6447, -24.0739) -> (1.9924, -22.773) construction
  line L356 (1.9924, -22.773) -> (2.0511, -22.0366) construction
  line L357 (2.0511, -22.0366) -> (2.0328, -21.8107) construction
  spline S114 degree 4 poles (2.0511, -22.0366) (2.0328, -21.8107) (2.0352, -21.5841) (2.0429, -21.3446) (2.1976, -21.1615) knots 1 1 1 1 1 2 2 2 2 2
  line L358 (2.0328, -21.8107) -> (2.0352, -21.5841) construction
  line L359 (2.0352, -21.5841) -> (2.0429, -21.3446) construction
  line L360 (2.0429, -21.3446) -> (2.1976, -21.1615) construction
  arc A61 (2.1976, -21.1615) -> (2.777, -21.0933) centre (0, 0) ccw
  arc A62 (2.777, -21.0933) -> (3.3543, -21.0092) centre (0, 0) ccw
  spline S115 degree 4 poles (3.7222, -21.8166) (3.6815, -21.5937) (3.6205, -21.3754) (3.5511, -21.146) (3.3543, -21.0092) knots 1 1 1 1 1 2 2 2 2 2
  line L361 (3.7222, -21.8166) -> (3.6815, -21.5937) construction
  line L362 (3.6815, -21.5937) -> (3.6205, -21.3754) construction
  line L363 (3.6205, -21.3754) -> (3.5511, -21.146) construction
  line L364 (3.5511, -21.146) -> (3.3543, -21.0092) construction
  line L365 (8.6834, -22.5134) -> (7.8186, -21.4814) construction
  spline S116 degree 2 poles (8.6834, -22.5134) (7.8186, -21.4814) (7.4541, -20.8388) knots 1 1 1 2 2 2
  line L366 (7.8186, -21.4814) -> (7.4541, -20.8388) construction
  spline S117 degree 2 poles (5.8001, -23.4225) (5.9166, -22.0811) (5.8466, -21.3456) knots 1 1 1 2 2 2
  line L367 (5.8001, -23.4225) -> (5.9166, -22.0811) construction
  line L368 (5.9166, -22.0811) -> (5.8466, -21.3456) construction
  line L369 (5.8466, -21.3456) -> (5.7894, -21.1264) construction
  spline S118 degree 4 poles (5.8466, -21.3456) (5.7894, -21.1264) (5.7524, -20.9028) (5.7183, -20.6656) (5.8389, -20.4584) knots 1 1 1 1 1 2 2 2 2 2
  line L370 (5.7894, -21.1264) -> (5.7524, -20.9028) construction
  line L371 (5.7524, -20.9028) -> (5.7183, -20.6656) construction
  line L372 (5.7183, -20.6656) -> (5.8389, -20.4584) construction
  arc A63 (5.8389, -20.4584) -> (6.3976, -20.2906) centre (0, 0) ccw
  arc A64 (6.3976, -20.2906) -> (6.9515, -20.1076) centre (0, 0) ccw
  spline S119 degree 4 poles (7.4541, -20.8388) (7.3752, -20.6264) (7.2773, -20.422) (7.1691, -20.2081) (6.9515, -20.1076) knots 1 1 1 1 1 2 2 2 2 2
  line L373 (7.4541, -20.8388) -> (7.3752, -20.6264) construction
  line L374 (7.3752, -20.6264) -> (7.2773, -20.422) construction
  line L375 (7.2773, -20.422) -> (7.1691, -20.2081) construction
  line L376 (7.1691, -20.2081) -> (6.9515, -20.1076) construction
  line L377 (12.4609, -20.6635) -> (11.43, -19.7973) construction
  spline S120 degree 2 poles (12.4609, -20.6635) (11.43, -19.7973) (10.9595, -19.2278) knots 1 1 1 2 2 2
  line L378 (11.43, -19.7973) -> (10.9595, -19.2278) construction
  spline S121 degree 2 poles (9.7793, -22.0595) (9.6611, -20.7182) (9.4644, -20.0061) knots 1 1 1 2 2 2
  line L379 (9.7793, -22.0595) -> (9.6611, -20.7182) construction
  line L380 (9.6611, -20.7182) -> (9.4644, -20.0061) construction
  line L381 (9.4644, -20.0061) -> (9.37, -19.8001) construction
  spline S122 degree 4 poles (9.4644, -20.0061) (9.37, -19.8001) (9.2947, -19.5864) (9.2199, -19.3586) (9.3027, -19.1337) knots 1 1 1 1 1 2 2 2 2 2
  line L382 (9.37, -19.8001) -> (9.2947, -19.5864) construction
  line L383 (9.2947, -19.5864) -> (9.2199, -19.3586) construction
  line L384 (9.2199, -19.3586) -> (9.3027, -19.1337) construction
  arc A65 (9.3027, -19.1337) -> (9.8238, -18.8714) centre (0, 0) ccw
  arc A66 (9.8238, -18.8714) -> (10.3376, -18.595) centre (0, 0) ccw
  spline S123 degree 4 poles (10.9595, -19.2278) (10.8449, -19.0323) (10.713, -18.8481) (10.5693, -18.6562) (10.3376, -18.595) knots 1 1 1 1 1 2 2 2 2 2
  line L385 (10.9595, -19.2278) -> (10.8449, -19.0323) construction
  line L386 (10.8449, -19.0323) -> (10.713, -18.8481) construction
  line L387 (10.713, -18.8481) -> (10.5693, -18.6562) construction
  line L388 (10.5693, -18.6562) -> (10.3376, -18.595) construction
  line L389 (15.8598, -18.1858) -> (14.6941, -17.5118) construction
  spline S124 degree 2 poles (15.8598, -18.1858) (14.6941, -17.5118) (14.1319, -17.0326) knots 1 1 1 2 2 2
  line L390 (14.6941, -17.5118) -> (14.1319, -17.0326) construction
  spline S125 degree 2 poles (13.4613, -20.0262) (13.112, -18.7258) (12.7946, -18.0587) knots 1 1 1 2 2 2
  line L391 (13.4613, -20.0262) -> (13.112, -18.7258) construction
  line L392 (13.112, -18.7258) -> (12.7946, -18.0587) construction
  line L393 (12.7946, -18.0587) -> (12.6659, -17.8722) construction
  spline S126 degree 4 poles (12.7946, -18.0587) (12.6659, -17.8722) (12.5546, -17.6748) (12.4415, -17.4635) (12.4839, -17.2276) knots 1 1 1 1 1 2 2 2 2 2
  line L394 (12.6659, -17.8722) -> (12.5546, -17.6748) construction
  line L395 (12.5546, -17.6748) -> (12.4415, -17.4635) construction
  line L396 (12.4415, -17.4635) -> (12.4839, -17.2276) construction
  arc A67 (12.4839, -17.2276) -> (12.9516, -16.8788) centre (0, 0) ccw
  arc A68 (12.9516, -16.8788) -> (13.4095, -16.5174) centre (0, 0) ccw
  spline S127 degree 4 poles (14.1319, -17.0326) (13.9851, -16.86) (13.8232, -16.7014) (13.6484, -16.5374) (13.4095, -16.5174) knots 1 1 1 1 1 2 2 2 2 2
  line L397 (14.1319, -17.0326) -> (13.9851, -16.86) construction
  line L398 (13.9851, -16.86) -> (13.8232, -16.7014) construction
  line L399 (13.8232, -16.7014) -> (13.6484, -16.5374) construction
  line L400 (13.6484, -16.5374) -> (13.4095, -16.5174) construction
  line L401 (18.7768, -15.1555) -> (17.5118, -14.6941) construction
  spline S128 degree 2 poles (18.7768, -15.1555) (17.5118, -14.6941) (16.8748, -14.3199) knots 1 1 1 2 2 2
  line L402 (17.5118, -14.6941) -> (16.8748, -14.3199) construction
  spline S129 degree 2 poles (16.7343, -17.3845) (16.1645, -16.1645) (15.7361, -15.5626) knots 1 1 1 2 2 2
  line L403 (16.7343, -17.3845) -> (16.1645, -16.1645) construction
  line L404 (16.1645, -16.1645) -> (15.7361, -15.5626) construction
  line L405 (15.7361, -15.5626) -> (15.5769, -15.4013) construction
  spline S130 degree 4 poles (15.7361, -15.5626) (15.5769, -15.4013) (15.4331, -15.2262) (15.2849, -15.0378) (15.2858, -14.7981) knots 1 1 1 1 1 2 2 2 2 2
  line L406 (15.5769, -15.4013) -> (15.4331, -15.2262) construction
  line L407 (15.4331, -15.2262) -> (15.2849, -15.0378) construction
  line L408 (15.2849, -15.0378) -> (15.2858, -14.7981) construction
  arc A69 (15.2858, -14.7981) -> (15.6858, -14.3734) centre (0, 0) ccw
  arc A70 (15.6858, -14.3734) -> (16.074, -13.9379) centre (0, 0) ccw
  spline S131 degree 4 poles (16.8748, -14.3199) (16.7003, -14.1753) (16.5133, -14.0473) (16.3127, -13.9162) (16.074, -13.9379) knots 1 1 1 1 1 2 2 2 2 2
  line L409 (16.8748, -14.3199) -> (16.7003, -14.1753) construction
  line L410 (16.7003, -14.1753) -> (16.5133, -14.0473) construction
  line L411 (16.5133, -14.0473) -> (16.3127, -13.9162) construction
  line L412 (16.3127, -13.9162) -> (16.074, -13.9379) construction
  line L413 (21.1233, -11.6647) -> (19.7973, -11.43) construction
  spline S132 degree 2 poles (21.1233, -11.6647) (19.7973, -11.43) (19.1051, -11.172) knots 1 1 1 2 2 2
  line L414 (19.7973, -11.43) -> (19.1051, -11.172) construction
  spline S133 degree 2 poles (19.4989, -14.2145) (18.7258, -13.112) (18.1995, -12.5936) knots 1 1 1 2 2 2
  line L415 (19.4989, -14.2145) -> (18.7258, -13.112) construction
  line L416 (18.7258, -13.112) -> (18.1995, -12.5936) construction
  line L417 (18.1995, -12.5936) -> (18.0147, -12.4624) construction